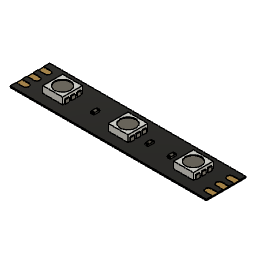
m v1 (Autodesk Fusion 360 design; units mm, degrees)
Autodesk Fusion 360 part; units mm, degrees
sketch "Sketch7" plane through (0, 0, 0) normal (0, 0, 1) x (1, 0, 0)
  line L0 (0, 0) -> (49.62, 0)
  line L1 (49.62, 0) -> (49.62, 10)
  line L2 (49.62, 10) -> (0, 10)
  line L3 (0, 10) -> (0, 0)
  line L4 (0, 10) -> (8.27, 10) construction
  line L5 (8.27, 10) -> (8.27, 0) construction
  line L6 (0, 5) -> (49.62, 5) construction
  line L7 (10.77, 2.5) -> (5.77, 2.5)
  line L8 (5.77, 2.5) -> (5.77, 7.5)
  line L9 (5.77, 7.5) -> (10.77, 7.5)
  line L10 (10.77, 7.5) -> (10.77, 2.5)
  line L11 (10.77, 2.5) -> (5.77, 7.5) construction
  line L12 (5.77, 2.5) -> (10.77, 7.5) construction
  line L13 (8.27, 5) -> (24.81, 5) construction
  line L14 (27.31, 2.5) -> (22.31, 2.5)
  line L15 (22.31, 2.5) -> (22.31, 7.5)
  line L16 (22.31, 7.5) -> (27.31, 7.5)
  line L17 (27.31, 7.5) -> (27.31, 2.5)
  line L18 (27.31, 2.5) -> (22.31, 7.5) construction
  line L19 (22.31, 2.5) -> (27.31, 7.5) construction
  line L20 (24.81, 5) -> (41.35, 5) construction
  line L21 (43.85, 2.5) -> (38.85, 2.5)
  line L22 (38.85, 2.5) -> (38.85, 7.5)
  line L23 (38.85, 7.5) -> (43.85, 7.5)
  line L24 (43.85, 7.5) -> (43.85, 2.5)
  line L25 (43.85, 2.5) -> (38.85, 7.5) construction
  line L26 (38.85, 2.5) -> (43.85, 7.5) construction
  point P0 (8.27, 5)
  point P1 (24.81, 5)
  point P2 (41.35, 5)
  dimension "d27" = 49.62
  dimension "d28" = 10
  dimension "d29" = 8.27
  dimension "d30" = 5
  dimension "d31" = 5
  dimension "d32" = 16.54
  dimension "d33" = 5
  dimension "d34" = 5
  dimension "d35" = 16.54
  dimension "d36" = 5
  dimension "d37" = 5
  constraint coincident L0.start L3.end
  constraint horizontal L0
  constraint perpendicular L0 L1
  constraint perpendicular L1 L2
  constraint perpendicular L0 L3
  constraint perpendicular L3 L4
  constraint coincident L0 L5.end
  constraint perpendicular L0 L5
  constraint midpoint L3 L6.start
  constraint midpoint L1 L6.end
  constraint horizontal L7
  constraint perpendicular L7 L8
  constraint parallel L7 L9
  constraint parallel L8 L10
  constraint coincident L11 P0
  constraint coincident L12 P0
  constraint midpoint L5 P0
  constraint coincident P0 L13.start
  constraint parallel L6 L13
  constraint horizontal L14
  constraint perpendicular L14 L15
  constraint parallel L14 L16
  constraint parallel L15 L17
  constraint coincident L18 P1
  constraint coincident L19 P1
  constraint coincident P1 L13.end
  constraint parallel L6 L20
  constraint horizontal L21
  constraint perpendicular L21 L22
  constraint parallel L21 L23
  constraint parallel L22 L24
  constraint coincident L25 P2
  constraint coincident L26 P2
  constraint coincident P2 L20.end
  measures "d27" distance of L0.start L0.end
  measures "d28" distance of L0.end L1.end
  measures "d29" distance of L2.end L4.end
  measures "d30" distance of L8.end L9.end
  measures "d31" distance of L7.end L8.end
  measures "d32" distance of P0 P1
  measures "d33" distance of L15.end L16.end
  measures "d34" distance of L14.end L15.end
  measures "d35" distance of P1 P2
  measures "d36" distance of L22.end L23.end
  measures "d37" distance of L21.end L22.end
extrude "Extrude4" add sketch "Sketch7" along normal blind 2 contours L7 L8 L9 L10 | L14 L15 L16 L17 | L21 L22 L23 L24 makes body 1 at (25.6433, 4.1667, 0) makes body 2 at (9.1033, 4.1667, 0) makes body 3 at (42.1833, 4.1667, 0)
extrude "Extrude3" add sketch "Sketch7" along normal blind 0.3 separate body makes body 4
sketch "Sketch8" plane through (0, 0, 2) normal (0, 0, 1) x (-1, 0, 0)
  line L0 (-10.77, -7.5) -> (-5.77, -7.5)
  line L1 (-5.77, -7.5) -> (-5.77, -2.5)
  line L2 (-5.77, -2.5) -> (-10.77, -2.5)
  line L3 (-10.77, -2.5) -> (-10.77, -7.5)
  circle A0 centre (-8.27, -5) radius 2
  circle A1 centre (-24.81, -5) radius 2
  circle A2 centre (-41.35, -5) radius 2
  point P0 (-8.27, -5)
  point P1 (-24.81, -5)
  point P2 (-41.35, -5)
  dimension "d42" = 4
  dimension "d43" = 4
  dimension "d44" = 4
  constraint coincident P0 A0.centre
  constraint coincident P1 A1.centre
  constraint coincident P2 A2.centre
  measures "d42" diameter of A0
  measures "d43" diameter of A1
  measures "d44" diameter of A2
extrude "Extrude5" cut sketch "Sketch8" against normal blind 0.2 contours A0 | A1 | A2 bodies 1 2 3
sketch "Sketch9" plane through (0, 0, 0.3) normal (0, 0, 1) x (-1, 0, 0)
  line L0 (-5.77, -7.5) -> (-10.77, -7.5)
  line L1 (-10.77, -7.5) -> (-10.77, -2.5)
  line L2 (-10.77, -2.5) -> (-5.77, -2.5)
  line L3 (-5.77, -2.5) -> (-5.77, -7.5)
  line L4 (-38.85, -7.5) -> (-43.85, -7.5)
  line L5 (-43.85, -7.5) -> (-43.85, -2.5)
  line L6 (-43.85, -2.5) -> (-38.85, -2.5)
  line L7 (-38.85, -2.5) -> (-38.85, -7.5)
  line L8 (-22.31, -7.5) -> (-27.31, -7.5)
  line L9 (-27.31, -7.5) -> (-27.31, -2.5)
  line L10 (-27.31, -2.5) -> (-22.31, -2.5)
  line L11 (-22.31, -2.5) -> (-22.31, -7.5)
  line L12 (0, -10) -> (0, 0)
  line L13 (0, 0) -> (-49.62, 0)
  line L14 (-49.62, 0) -> (-49.62, -10)
  line L15 (-49.62, -10) -> (0, -10)
  line L16 (-5.77, -7.5) -> (-5.77, -7) construction
  line L17 (-5.77, -7) -> (-5.77, -6)
  line L18 (-5.77, -6) -> (-5.77, -5.5) construction
  line L19 (-5.77, -5.5) -> (-5.77, -4.5)
  line L20 (-5.77, -4.5) -> (-5.77, -4) construction
  line L21 (-5.77, -4) -> (-5.77, -3) construction
  line L22 (-5.77, -3) -> (-5.77, -2.5) construction
  line L23 (-5.77, -7) -> (-5.57, -7)
  line L24 (-5.77, -6) -> (-5.57, -6)
  line L25 (-5.57, -6) -> (-5.57, -7)
  line L26 (-5.77, -5.5) -> (-5.57, -5.5)
  line L27 (-5.57, -5.5) -> (-5.57, -4.5)
  line L28 (-5.57, -4.5) -> (-5.77, -4.5)
  line L29 (-5.77, -3) -> (-5.57, -3)
  line L30 (-5.57, -3) -> (-5.57, -4)
  line L31 (-5.57, -4) -> (-5.77, -4)
  dimension "d47" = 0.5
  dimension "d48" = 1
  dimension "d49" = 0.5
  dimension "d50" = 1
  dimension "d51" = 0.5
  dimension "d52" = 1
  dimension "d53" = 0.2
  dimension "d54" = 0.2
  constraint coincident L0.start L3.end
  constraint perpendicular L0 L16
  constraint parallel L3 L17
  constraint parallel L3 L18
  constraint parallel L18 L19
  constraint parallel L3 L20
  constraint parallel L3 L21
  constraint coincident L2.end L3.start
  constraint perpendicular L16 L23
  constraint perpendicular L17 L24
  constraint perpendicular L18 L26
  constraint perpendicular L26 L27
  constraint perpendicular L22 L29
  constraint perpendicular L29 L30
  measures "d47" distance of L0.start L16.end
  measures "d48" distance of L16.end L17.end
  measures "d49" distance of L17.end L18.end
  measures "d50" distance of L18.end L19.end
  measures "d51" distance of L19.end L20.end
  measures "d52" distance of L20.end L21.end
  measures "d53" distance of L16.end L23.end
  measures "d54" distance of L17.end L24.end
extrude "Extrude6" add sketch "Sketch9" along normal blind 1 contours L3 L17 L23 L24 L25 | L3 L19 L26 L27 L28 | L3 L29 L30 L31 bodies 2 4
sketch "Sketch10" plane through (0, 0, 0.3) normal (0, 0, 1) x (-1, 0, 0)
  line L0 (-5.77, -6) -> (-5.57, -6)
  line L1 (-5.57, -6) -> (-5.57, -7)
  line L2 (-5.57, -7) -> (-5.77, -7)
  line L3 (-5.77, -7) -> (-5.77, -7.5)
  line L4 (-5.77, -7.5) -> (-10.77, -7.5)
  line L5 (-10.77, -7.5) -> (-10.77, -2.5)
  line L6 (-10.77, -2.5) -> (-5.77, -2.5)
  line L7 (-5.77, -2.5) -> (-5.77, -3)
  line L8 (-5.77, -3) -> (-5.57, -3)
  line L9 (-5.57, -3) -> (-5.57, -4)
  line L10 (-5.57, -4) -> (-5.77, -4)
  line L11 (-5.77, -4) -> (-5.77, -4.5)
  line L12 (-5.77, -4.5) -> (-5.57, -4.5)
  line L13 (-5.57, -4.5) -> (-5.57, -5.5)
  line L14 (-5.57, -5.5) -> (-5.77, -5.5)
  line L15 (-5.77, -5.5) -> (-5.77, -6)
  line L16 (-38.85, -7.5) -> (-43.85, -7.5)
  line L17 (-43.85, -7.5) -> (-43.85, -2.5)
  line L18 (-43.85, -2.5) -> (-38.85, -2.5)
  line L19 (-38.85, -2.5) -> (-38.85, -7.5)
  line L20 (-22.31, -7.5) -> (-27.31, -7.5)
  line L21 (-27.31, -7.5) -> (-27.31, -2.5)
  line L22 (-27.31, -2.5) -> (-22.31, -2.5)
  line L23 (-22.31, -2.5) -> (-22.31, -7.5)
  line L24 (0, -10) -> (0, 0)
  line L25 (0, 0) -> (-49.62, 0)
  line L26 (-49.62, 0) -> (-49.62, -10)
  line L27 (-49.62, -10) -> (0, -10)
  line L28 (-5.77, -6) -> (-10.77, -6) construction
  line L29 (-5.77, -4.5) -> (-10.77, -4.5) construction
  line L30 (-5.77, -3) -> (-10.77, -3) construction
  line L31 (-5.77, -4) -> (-10.77, -4) construction
  line L32 (-5.77, -5.5) -> (-10.77, -5.5) construction
  line L33 (-5.77, -7) -> (-10.77, -7) construction
  line L34 (-10.77, -7) -> (-10.97, -7)
  line L35 (-10.97, -7) -> (-10.97, -3) construction
  line L36 (-10.97, -3) -> (-10.77, -3)
  line L37 (-10.77, -4) -> (-10.97, -4)
  line L38 (-10.97, -4) -> (-10.97, -3)
  line L39 (-10.77, -4.5) -> (-10.97, -4.5)
  line L40 (-10.97, -4.5) -> (-10.97, -5.5)
  line L41 (-10.77, -5.5) -> (-10.97, -5.5)
  line L42 (-10.77, -6) -> (-10.97, -6)
  line L43 (-10.97, -6) -> (-10.97, -7)
  line L44 (-10.97, -3) -> (-43.85, -3) construction
  line L45 (-43.85, -3) -> (-44.05, -3) construction
  line L46 (-10.97, -4) -> (-43.85, -4) construction
  line L47 (-44.05, -7) -> (-10.77, -7) construction
  line L48 (-10.97, -6) -> (-44.8, -6) construction
  line L49 (-10.97, -5.5) -> (-44.05, -5.5) construction
  line L50 (-10.77, -4.5) -> (-44.05, -4.5) construction
  line L51 (-22.31, -3) -> (-22.11, -3) construction
  line L52 (-22.11, -3) -> (-22.11, -7) construction
  line L53 (-27.31, -7) -> (-27.51, -7) construction
  line L54 (-27.51, -7) -> (-27.51, -3) construction
  line L55 (-27.31, -3) -> (-27.51, -3) construction
  line L56 (-43.85, -7) -> (-44.05, -7)
  line L57 (-43.85, -7) -> (-43.85, -3)
  line L58 (-43.85, -3) -> (-44.05, -3)
  line L59 (-43.85, -4) -> (-44.05, -4)
  line L60 (-43.85, -4.5) -> (-44.05, -4.5)
  line L61 (-43.85, -5.5) -> (-44.05, -5.5)
  line L62 (-43.85, -6.004) -> (-44.05, -6)
  line L63 (-38.85, -3) -> (-38.65, -3)
  line L64 (-38.65, -7) -> (-38.85, -7)
  line L65 (-38.85, -3) -> (-38.85, -7)
  line L66 (-38.65, -6) -> (-38.85, -6)
  line L67 (-38.65, -5.5) -> (-38.85, -5.5)
  line L68 (-38.65, -4.5) -> (-38.85, -4.5028)
  line L69 (-38.65, -4) -> (-38.85, -3.9993)
  line L70 (-38.65, -3) -> (-38.65, -4)
  line L71 (-38.65, -4.5) -> (-38.65, -5.5)
  line L72 (-38.65, -6) -> (-38.65, -7)
  line L73 (-44.05, -3) -> (-44.05, -4)
  line L74 (-44.05, -4.5) -> (-44.05, -5.5)
  line L75 (-44.05, -6) -> (-44.05, -7)
  line L76 (-27.31, -3) -> (-27.51, -3)
  line L77 (-27.51, -3) -> (-27.51, -4)
  line L78 (-27.51, -4) -> (-27.31, -4)
  line L79 (-27.31, -4.5) -> (-27.51, -4.5)
  line L80 (-27.51, -4.5) -> (-27.51, -5.5)
  line L81 (-27.51, -5.5) -> (-27.3, -5.5)
  line L82 (-27.31, -6) -> (-27.51, -6)
  line L83 (-27.51, -6) -> (-27.51, -7)
  line L84 (-27.51, -7) -> (-27.31, -7)
  line L85 (-22.31, -7) -> (-22.11, -7)
  line L86 (-22.11, -6) -> (-22.11, -7)
  line L87 (-22.11, -6) -> (-22.31, -6)
  line L88 (-22.11, -5.5) -> (-22.31, -5.5)
  line L89 (-22.11, -5.5) -> (-22.11, -4.5)
  line L90 (-22.31, -4.5) -> (-22.11, -4.5)
  line L91 (-22.11, -4) -> (-22.31, -4)
  line L92 (-22.11, -4) -> (-22.11, -3)
  line L93 (-22.11, -3) -> (-22.31, -3)
  dimension "d57" = 0.2
  dimension "d60" = 32.88
  dimension "d61" = 0.2
  dimension "d62" = 4
  dimension "d63" = 0.2
  dimension "d64" = 0.2
  dimension "d65" = 0.2
  constraint coincident L0.start L15.end
  constraint coincident L5 L28.end
  constraint perpendicular L5 L28
  constraint coincident L11.end L12.start
  constraint coincident L5 L29.end
  constraint perpendicular L5 L29
  constraint coincident L7.end L8.start
  constraint coincident L5 L30.end
  constraint perpendicular L5 L30
  constraint coincident L10.end L11.start
  constraint coincident L5 L31.end
  constraint perpendicular L5 L31
  constraint coincident L14.end L15.start
  constraint coincident L5 L32.end
  constraint perpendicular L5 L32
  constraint coincident L2.end L3.start
  constraint coincident L5 L33.end
  constraint perpendicular L5 L33
  constraint perpendicular L5 L34
  constraint perpendicular L34 L35
  constraint coincident L35 L37.end
  constraint perpendicular L35 L37
  constraint coincident L35 L39.end
  constraint perpendicular L35 L39
  constraint coincident L35 L40.end
  constraint coincident L35 L42.end
  constraint perpendicular L35 L42
  constraint coincident L17 L44.end
  constraint perpendicular L17 L44
  constraint horizontal L45
  constraint coincident L17 L46.end
  constraint perpendicular L17 L46
  constraint perpendicular L17 L48
  constraint coincident L44 L51.start
  constraint coincident L23 L51.start
  constraint perpendicular L23 L51
  constraint coincident L47 L52.end
  constraint perpendicular L47 L52
  constraint coincident L47 L53.start
  constraint coincident L21 L53.start
  constraint perpendicular L21 L53
  constraint coincident L44 L54.end
  constraint perpendicular L44 L54
  constraint coincident L44 L55.start
  constraint coincident L21 L55.start
  constraint coincident L47 L56.start
  constraint coincident L17 L56.start
  constraint coincident L57 L60.start
  constraint coincident L50 L60.start
  constraint coincident L57 L61.start
  constraint coincident L49 L61.start
  constraint coincident L57 L62.start
  constraint coincident L48 L62.end
  constraint coincident L44 L63.start
  constraint coincident L19 L63.start
  constraint perpendicular L19 L63
  constraint coincident L47 L64.start
  constraint coincident L47 L64.end
  constraint coincident L19 L64.end
  constraint coincident L48 L66.start
  constraint coincident L48 L66.end
  constraint coincident L19 L66.end
  constraint coincident L49 L67.start
  constraint coincident L65 L67.end
  constraint coincident L49 L67.end
  constraint coincident L50 L68.start
  constraint coincident L65 L68.end
  constraint coincident L46 L69.start
  constraint coincident L65 L69.end
  constraint parallel L70 L71
  constraint perpendicular L64 L72
  constraint perpendicular L59 L73
  constraint perpendicular L61 L74
  constraint parallel L74 L75
  constraint coincident L54 L77.end
  constraint coincident L46 L77.end
  constraint coincident L46 L78.end
  constraint coincident L21 L78.end
  constraint coincident L50 L79.start
  constraint coincident L21 L79.start
  constraint coincident L54 L79.end
  constraint coincident L50 L79.end
  constraint perpendicular L54 L79
  constraint midpoint L49 L80.end
  constraint perpendicular L49 L80
  constraint coincident L49 L81.end
  constraint perpendicular L80 L81
  constraint coincident L48 L82.start
  constraint coincident L21 L82.start
  constraint coincident L54 L82.end
  constraint coincident L48 L82.end
  constraint coincident L47 L85.start
  constraint coincident L23 L85.start
  constraint coincident L52 L86.start
  constraint coincident L48 L86.start
  constraint coincident L48 L87.end
  constraint coincident L23 L87.end
  constraint coincident L52 L88.start
  constraint coincident L49 L88.start
  constraint coincident L49 L88.end
  constraint coincident L23 L88.end
  constraint perpendicular L23 L88
  constraint coincident L52 L89.end
  constraint coincident L50 L89.end
  constraint coincident L50 L90.start
  constraint coincident L23 L90.start
  constraint perpendicular L89 L90
  constraint coincident L46 L91.start
  constraint coincident L52 L91.start
  constraint coincident L46 L91.end
  constraint coincident L23 L91.end
  measures "d57" distance of L33.end L34.end
  measures "d60" distance of L35.end L44.end
  measures "d61" distance of L44.end L45.end
  measures "d62" distance of L45.end L47.start
  measures "d63" distance of L51.start L51.end
  measures "d64" distance of L53.start L53.end
  measures "d65" distance of L63.start L63.end
extrude "Extrude7" add sketch "Sketch10" along normal blind 1 contours L5 L34 L42 L43 | L5 L39 L40 L41 | L5 L36 L37 L38 | L19 L64 L65 L66 L72 | L17 L56 L57 L62 L75 | L19 L65 L67 L68 L71 | L17 L57 L60 L61 L74 | L19 L63 L65 L69 L70 | L17 L57 L58 L59 L73 | L23 L85 L86 L87 | L21 L82 L83 L84 | L23 L88 L89 L90 | L21 L79 L80 L81 | L23 L91 L92 L93 | L21 L76 L77 L78 bodies 1 2 3
sketch "Sketch11" plane through (0, 0, 0.3) normal (0, 0, 1) x (-1, 0, 0)
  line L0 (-44.05, -3) -> (-43.85, -3)
  line L1 (-43.85, -3) -> (-43.85, -2.5)
  line L2 (-43.85, -2.5) -> (-38.85, -2.5)
  line L3 (-38.85, -2.5) -> (-38.85, -3)
  line L4 (-38.85, -3) -> (-38.65, -3)
  line L5 (-38.65, -3) -> (-38.65, -4)
  line L6 (-38.65, -4) -> (-38.85, -3.9993)
  line L7 (-38.85, -3.9993) -> (-38.85, -4.5028)
  line L8 (-38.85, -4.5028) -> (-38.65, -4.5)
  line L9 (-38.65, -4.5) -> (-38.65, -5.5)
  line L10 (-38.65, -5.5) -> (-38.85, -5.5)
  line L11 (-38.85, -5.5) -> (-38.85, -6)
  line L12 (-38.85, -6) -> (-38.65, -6)
  line L13 (-38.65, -6) -> (-38.65, -7)
  line L14 (-38.65, -7) -> (-38.85, -7)
  line L15 (-38.85, -7) -> (-38.85, -7.5)
  line L16 (-38.85, -7.5) -> (-43.85, -7.5)
  line L17 (-43.85, -7.5) -> (-43.85, -7)
  line L18 (-43.85, -7) -> (-44.05, -7)
  line L19 (-44.05, -7) -> (-44.05, -6)
  line L20 (-44.05, -6) -> (-43.85, -6.004)
  line L21 (-43.85, -6.004) -> (-43.85, -5.5)
  line L22 (-43.85, -5.5) -> (-44.05, -5.5)
  line L23 (-44.05, -5.5) -> (-44.05, -4.5)
  line L24 (-44.05, -4.5) -> (-43.85, -4.5)
  line L25 (-43.85, -4.5) -> (-43.85, -4)
  line L26 (-43.85, -4) -> (-44.05, -4)
  line L27 (-44.05, -4) -> (-44.05, -3)
  line L28 (-27.51, -6) -> (-27.31, -6)
  line L29 (-27.31, -6) -> (-27.31, -5.5)
  line L30 (-27.31, -5.5) -> (-27.51, -5.5)
  line L31 (-27.51, -5.5) -> (-27.51, -4.5)
  line L32 (-27.51, -4.5) -> (-27.31, -4.5)
  line L33 (-27.31, -4.5) -> (-27.31, -4)
  line L34 (-27.31, -4) -> (-27.51, -4)
  line L35 (-27.51, -4) -> (-27.51, -3)
  line L36 (-27.51, -3) -> (-27.31, -3)
  line L37 (-27.31, -3) -> (-27.31, -2.5)
  line L38 (-27.31, -2.5) -> (-22.31, -2.5)
  line L39 (-22.31, -2.5) -> (-22.31, -3)
  line L40 (-22.31, -3) -> (-22.11, -3)
  line L41 (-22.11, -3) -> (-22.11, -4)
  line L42 (-22.11, -4) -> (-22.31, -4)
  line L43 (-22.31, -4) -> (-22.31, -4.5)
  line L44 (-22.31, -4.5) -> (-22.11, -4.5)
  line L45 (-22.11, -4.5) -> (-22.11, -5.5)
  line L46 (-22.11, -5.5) -> (-22.31, -5.5)
  line L47 (-22.31, -5.5) -> (-22.31, -6)
  line L48 (-22.31, -6) -> (-22.11, -6)
  line L49 (-22.11, -6) -> (-22.11, -7)
  line L50 (-22.11, -7) -> (-22.31, -7)
  line L51 (-22.31, -7) -> (-22.31, -7.5)
  line L52 (-22.31, -7.5) -> (-27.31, -7.5)
  line L53 (-27.31, -7.5) -> (-27.31, -7)
  line L54 (-27.31, -7) -> (-27.51, -7)
  line L55 (-27.51, -7) -> (-27.51, -6)
  line L56 (0, -10) -> (0, 0)
  line L57 (0, 0) -> (-49.62, 0)
  line L58 (-49.62, 0) -> (-49.62, -10)
  line L59 (-49.62, -10) -> (0, -10)
  line L60 (-10.77, -5.5) -> (-10.97, -5.5)
  line L61 (-10.97, -5.5) -> (-10.97, -4.5)
  line L62 (-10.97, -4.5) -> (-10.77, -4.5)
  line L63 (-10.77, -4.5) -> (-10.77, -4)
  line L64 (-10.77, -4) -> (-10.97, -4)
  line L65 (-10.97, -4) -> (-10.97, -3)
  line L66 (-10.97, -3) -> (-10.77, -3)
  line L67 (-10.77, -3) -> (-10.77, -2.5)
  line L68 (-10.77, -2.5) -> (-5.77, -2.5)
  line L69 (-5.77, -2.5) -> (-5.77, -3)
  line L70 (-5.77, -3) -> (-5.57, -3)
  line L71 (-5.57, -3) -> (-5.57, -4)
  line L72 (-5.57, -4) -> (-5.77, -4)
  line L73 (-5.77, -4) -> (-5.77, -4.5)
  line L74 (-5.77, -4.5) -> (-5.57, -4.5)
  line L75 (-5.57, -4.5) -> (-5.57, -5.5)
  line L76 (-5.57, -5.5) -> (-5.77, -5.5)
  line L77 (-5.77, -5.5) -> (-5.77, -6)
  line L78 (-5.77, -6) -> (-5.57, -6)
  line L79 (-5.57, -6) -> (-5.57, -7)
  line L80 (-5.57, -7) -> (-5.77, -7)
  line L81 (-5.77, -7) -> (-5.77, -7.5)
  line L82 (-5.77, -7.5) -> (-10.77, -7.5)
  line L83 (-10.77, -7.5) -> (-10.77, -7)
  line L84 (-10.77, -7) -> (-10.97, -7)
  line L85 (-10.97, -7) -> (-10.97, -6)
  line L86 (-10.97, -6) -> (-10.77, -6)
  line L87 (-10.77, -6) -> (-10.77, -5.5)
  line L88 (0, -5) -> (0, -5.75)
  line L89 (0, -5) -> (0, -4.25)
  line L90 (0, -4.25) -> (-2.5, -4.25)
  line L91 (-2.5, -4.25) -> (-2.5, -5.75)
  line L92 (-2.5, -5.75) -> (0, -5.75)
  line L93 (0, -4.25) -> (0, -3) construction
  line L94 (0, -3) -> (0, -1.5) construction
  line L95 (0, -1.5) -> (-2.5, -1.5)
  line L96 (-2.5, -1.5) -> (-2.5, -3)
  line L97 (-2.5, -3) -> (0, -3)
  line L98 (0, -5.75) -> (0, -7) construction
  line L99 (0, -7) -> (-2.5, -7)
  line L100 (-2.5, -7) -> (-2.5, -8.5)
  line L101 (-2.5, -8.5) -> (0, -8.5)
  line L102 (-2.5, -1.5) -> (-1.5, -1.5)
  line L103 (-2.5, -1.5) -> (-1.75, -1.5) construction
  line L104 (-1.75, -1.5) -> (-1.75, -3) construction
  circle A0 centre (-1.75, -2.25) radius 0.75
  line L105 (-1.75, -3) -> (-1.75, -8.5) construction
  line L106 (-1.75, -4.25) -> (-1.75, -5.75) construction
  line L107 (-1.75, -7) -> (-1.75, -8.5) construction
  circle A1 centre (-1.75, -5) radius 0.75
  circle A2 centre (-1.75, -7.75) radius 0.75
  dimension "d66" = 0.75
  dimension "d67" = 0.75
  dimension "d68" = 1.5
  dimension "d69" = 1.5
  dimension "d72" = 1
  dimension "d73" = 0.75
  dimension "d74" = 1.5
  dimension "d75" = 1.5
  dimension "d76" = 1.5
  constraint midpoint L56 L88.start
  constraint parallel L56 L88
  constraint parallel L88 L89
  constraint perpendicular L89 L90
  constraint perpendicular L90 L91
  constraint coincident L56 L93.end
  constraint perpendicular L90 L93
  constraint parallel L56 L94
  constraint perpendicular L94 L95
  constraint perpendicular L95 L96
  constraint perpendicular L93 L97
  constraint coincident L56 L98.end
  constraint perpendicular L56 L99
  constraint perpendicular L99 L100
  constraint coincident L56 L101.end
  constraint perpendicular L100 L101
  constraint perpendicular L96 L102
  constraint perpendicular L96 L103
  constraint coincident L97 L104.end
  constraint perpendicular L97 L104
  constraint midpoint L104 A0.centre
  constraint coincident L101 L105.end
  constraint perpendicular L101 L105
  constraint coincident L105 L106.start
  constraint coincident L90 L106.start
  constraint midpoint L105 L106.end
  constraint coincident L105 L107.start
  constraint coincident L99 L107.start
  constraint perpendicular L101 L107
  constraint midpoint L106 A1.centre
  constraint midpoint L107 A2.centre
  measures "d66" distance of L88.start L88.end
  measures "d67" distance of L88.start L89.end
  measures "d68" distance of L90.end L91.end
  measures "d69" distance of L93.end L94.end
  measures "d72" distance of L95.end L102.end
  measures "d73" distance of L95.end L103.end
  measures "d74" diameter of A0
  measures "d75" diameter of A1
  measures "d76" diameter of A2
sketch "Sketch13" plane through (0, 0, 0.3) normal (0, 0, 1) x (-1, 0, 0)
  line L0 (0, 0) -> (-49.62, 0)
  line L1 (-49.62, 0) -> (-49.62, -10)
  line L2 (-49.62, -10) -> (0, -10)
  line L3 (0, -10) -> (0, 0)
  line L4 (-44.05, -3) -> (-43.85, -3)
  line L5 (-43.85, -3) -> (-43.85, -2.5)
  line L6 (-43.85, -2.5) -> (-38.85, -2.5)
  line L7 (-38.85, -2.5) -> (-38.85, -3)
  line L8 (-38.85, -3) -> (-38.65, -3)
  line L9 (-38.65, -3) -> (-38.65, -4)
  line L10 (-38.65, -4) -> (-38.85, -3.9993)
  line L11 (-38.85, -3.9993) -> (-38.85, -4.5028)
  line L12 (-38.85, -4.5028) -> (-38.65, -4.5)
  line L13 (-38.65, -4.5) -> (-38.65, -5.5)
  line L14 (-38.65, -5.5) -> (-38.85, -5.5)
  line L15 (-38.85, -5.5) -> (-38.85, -6)
  line L16 (-38.85, -6) -> (-38.65, -6)
  line L17 (-38.65, -6) -> (-38.65, -7)
  line L18 (-38.65, -7) -> (-38.85, -7)
  line L19 (-38.85, -7) -> (-38.85, -7.5)
  line L20 (-38.85, -7.5) -> (-43.85, -7.5)
  line L21 (-43.85, -7.5) -> (-43.85, -7)
  line L22 (-43.85, -7) -> (-44.05, -7)
  line L23 (-44.05, -7) -> (-44.05, -6)
  line L24 (-44.05, -6) -> (-43.85, -6.004)
  line L25 (-43.85, -6.004) -> (-43.85, -5.5)
  line L26 (-43.85, -5.5) -> (-44.05, -5.5)
  line L27 (-44.05, -5.5) -> (-44.05, -4.5)
  line L28 (-44.05, -4.5) -> (-43.85, -4.5)
  line L29 (-43.85, -4.5) -> (-43.85, -4)
  line L30 (-43.85, -4) -> (-44.05, -4)
  line L31 (-44.05, -4) -> (-44.05, -3)
  line L32 (-27.51, -6) -> (-27.31, -6)
  line L33 (-27.31, -6) -> (-27.31, -5.5)
  line L34 (-27.31, -5.5) -> (-27.51, -5.5)
  line L35 (-27.51, -5.5) -> (-27.51, -4.5)
  line L36 (-27.51, -4.5) -> (-27.31, -4.5)
  line L37 (-27.31, -4.5) -> (-27.31, -4)
  line L38 (-27.31, -4) -> (-27.51, -4)
  line L39 (-27.51, -4) -> (-27.51, -3)
  line L40 (-27.51, -3) -> (-27.31, -3)
  line L41 (-27.31, -3) -> (-27.31, -2.5)
  line L42 (-27.31, -2.5) -> (-22.31, -2.5)
  line L43 (-22.31, -2.5) -> (-22.31, -3)
  line L44 (-22.31, -3) -> (-22.11, -3)
  line L45 (-22.11, -3) -> (-22.11, -4)
  line L46 (-22.11, -4) -> (-22.31, -4)
  line L47 (-22.31, -4) -> (-22.31, -4.5)
  line L48 (-22.31, -4.5) -> (-22.11, -4.5)
  line L49 (-22.11, -4.5) -> (-22.11, -5.5)
  line L50 (-22.11, -5.5) -> (-22.31, -5.5)
  line L51 (-22.31, -5.5) -> (-22.31, -6)
  line L52 (-22.31, -6) -> (-22.11, -6)
  line L53 (-22.11, -6) -> (-22.11, -7)
  line L54 (-22.11, -7) -> (-22.31, -7)
  line L55 (-22.31, -7) -> (-22.31, -7.5)
  line L56 (-22.31, -7.5) -> (-27.31, -7.5)
  line L57 (-27.31, -7.5) -> (-27.31, -7)
  line L58 (-27.31, -7) -> (-27.51, -7)
  line L59 (-27.51, -7) -> (-27.51, -6)
  line L60 (-10.77, -5.5) -> (-10.97, -5.5)
  line L61 (-10.97, -5.5) -> (-10.97, -4.5)
  line L62 (-10.97, -4.5) -> (-10.77, -4.5)
  line L63 (-10.77, -4.5) -> (-10.77, -4)
  line L64 (-10.77, -4) -> (-10.97, -4)
  line L65 (-10.97, -4) -> (-10.97, -3)
  line L66 (-10.97, -3) -> (-10.77, -3)
  line L67 (-10.77, -3) -> (-10.77, -2.5)
  line L68 (-10.77, -2.5) -> (-5.77, -2.5)
  line L69 (-5.77, -2.5) -> (-5.77, -3)
  line L70 (-5.77, -3) -> (-5.57, -3)
  line L71 (-5.57, -3) -> (-5.57, -4)
  line L72 (-5.57, -4) -> (-5.77, -4)
  line L73 (-5.77, -4) -> (-5.77, -4.5)
  line L74 (-5.77, -4.5) -> (-5.57, -4.5)
  line L75 (-5.57, -4.5) -> (-5.57, -5.5)
  line L76 (-5.57, -5.5) -> (-5.77, -5.5)
  line L77 (-5.77, -5.5) -> (-5.77, -6)
  line L78 (-5.77, -6) -> (-5.57, -6)
  line L79 (-5.57, -6) -> (-5.57, -7)
  line L80 (-5.57, -7) -> (-5.77, -7)
  line L81 (-5.77, -7) -> (-5.77, -7.5)
  line L82 (-5.77, -7.5) -> (-10.77, -7.5)
  line L83 (-10.77, -7.5) -> (-10.77, -7)
  line L84 (-10.77, -7) -> (-10.97, -7)
  line L85 (-10.97, -7) -> (-10.97, -6)
  line L86 (-10.97, -6) -> (-10.77, -6)
  line L87 (-10.77, -6) -> (-10.77, -5.5)
  line L88 (-49.62, -5) -> (-49.62, -4.25)
  line L89 (-49.62, -5) -> (-49.62, -5.75)
  line L90 (-49.62, -5.75) -> (-47.12, -5.75)
  line L91 (-47.12, -5.75) -> (-47.12, -4.25)
  line L92 (-47.12, -4.25) -> (-49.62, -4.25)
  line L93 (-49.62, -4.25) -> (-49.62, -3) construction
  line L94 (-49.62, -3) -> (-47.12, -3)
  line L95 (-47.12, -3) -> (-47.12, -1.5)
  line L96 (-47.12, -1.5) -> (-49.62, -1.5)
  line L97 (-49.62, -5.75) -> (-49.62, -7) construction
  line L98 (-49.62, -7) -> (-47.12, -7)
  line L99 (-47.12, -7) -> (-47.12, -8.5)
  line L100 (-47.12, -8.5) -> (-49.62, -8.5)
  line L101 (-47.12, -8.5) -> (-47.87, -8.5) construction
  line L102 (-47.87, -8.5) -> (-47.87, -1.5) construction
  line L103 (-47.87, -8.5) -> (-47.87, -7) construction
  line L104 (-47.87, -5.75) -> (-47.87, -4.4) construction
  line L105 (-47.87, -3) -> (-47.87, -1.5) construction
  circle A0 centre (-47.87, -7.75) radius 0.75
  circle A1 centre (-47.87, -5) radius 0.75
  circle A2 centre (-47.87, -2.25) radius 0.75
  dimension "d77" = 0.75
  dimension "d78" = 0.75
  dimension "d79" = 2.5
  dimension "d80" = 1.5
  dimension "d81" = 1.25
  dimension "d82" = 2.5
  dimension "d83" = 1.5
  dimension "d84" = 1.25
  dimension "d85" = 2.5
  dimension "d86" = 1.5
  dimension "d87" = 0.75
  dimension "d88" = 1.5
  dimension "d89" = 1.5
  dimension "d90" = 1.5
  constraint midpoint L1 L88.start
  constraint parallel L1 L88
  constraint parallel L1 L89
  constraint perpendicular L1 L90
  constraint perpendicular L90 L91
  constraint perpendicular L92 L93
  constraint perpendicular L93 L94
  constraint perpendicular L94 L95
  constraint coincident L1 L96.end
  constraint perpendicular L1 L96
  constraint perpendicular L90 L97
  constraint perpendicular L97 L98
  constraint perpendicular L98 L99
  constraint coincident L1 L100.end
  constraint perpendicular L1 L100
  constraint perpendicular L99 L101
  constraint coincident L96 L102.end
  constraint perpendicular L96 L102
  constraint coincident L98 L103.end
  constraint coincident L102 L103.end
  constraint coincident L90 L104.start
  constraint coincident L102 L104.start
  constraint coincident L102 L104.end
  constraint perpendicular L90 L104
  constraint coincident L102 L105.start
  constraint coincident L94 L105.start
  constraint midpoint L103 A0.centre
  constraint midpoint L102 A1.centre
  constraint midpoint L105 A2.centre
  measures "d77" distance of L88.start L88.end
  measures "d78" distance of L88.start L89.end
  measures "d79" distance of L89.end L90.end
  measures "d80" distance of L90.end L91.end
  measures "d81" distance of L88.end L93.end
  measures "d82" distance of L93.end L94.end
  measures "d83" distance of L94.end L95.end
  measures "d84" distance of L89.end L97.end
  measures "d85" distance of L97.end L98.end
  measures "d86" distance of L98.end L99.end
  measures "d87" distance of L99.end L101.end
  measures "d88" diameter of A0
  measures "d89" diameter of A1
  measures "d90" diameter of A2
extrude "Extrude8" cut sketch "Sketch11" sketch "Sketch13" against normal blind 0.1 contours L56 L99 L101 A2 | A2 | L56 L88 L89 L90 L92 A1 | A1 | L56 L95 L97 L102 A0 | A0 of sketch 2 contours L1 L94 L96 A2 | A2 | L1 L98 L100 A0 | L1 L88 L89 L90 L92 A1 | A0 | A1 bodies 1
sketch "Sketch14" plane through (0, 0, 0.3) normal (0, 0, 1) x (-1, 0, 0)
  line L0 (-10.77, -5.5) -> (-10.97, -5.5)
  line L1 (-10.97, -5.5) -> (-10.97, -4.5)
  line L2 (-10.97, -4.5) -> (-10.77, -4.5)
  line L3 (-10.77, -4.5) -> (-10.77, -4)
  line L4 (-10.77, -4) -> (-10.97, -4)
  line L5 (-10.97, -4) -> (-10.97, -3)
  line L6 (-10.97, -3) -> (-10.77, -3)
  line L7 (-10.77, -3) -> (-10.77, -2.5)
  line L8 (-10.77, -2.5) -> (-5.77, -2.5)
  line L9 (-5.77, -2.5) -> (-5.77, -3)
  line L10 (-5.77, -3) -> (-5.57, -3)
  line L11 (-5.57, -3) -> (-5.57, -4)
  line L12 (-5.57, -4) -> (-5.77, -4)
  line L13 (-5.77, -4) -> (-5.77, -4.5)
  line L14 (-5.77, -4.5) -> (-5.57, -4.5)
  line L15 (-5.57, -4.5) -> (-5.57, -5.5)
  line L16 (-5.57, -5.5) -> (-5.77, -5.5)
  line L17 (-5.77, -5.5) -> (-5.77, -6)
  line L18 (-5.77, -6) -> (-5.57, -6)
  line L19 (-5.57, -6) -> (-5.57, -7)
  line L20 (-5.57, -7) -> (-5.77, -7)
  line L21 (-5.77, -7) -> (-5.77, -7.5)
  line L22 (-5.77, -7.5) -> (-10.77, -7.5)
  line L23 (-10.77, -7.5) -> (-10.77, -7)
  line L24 (-10.77, -7) -> (-10.97, -7)
  line L25 (-10.97, -7) -> (-10.97, -6)
  line L26 (-10.97, -6) -> (-10.77, -6)
  line L27 (-10.77, -6) -> (-10.77, -5.5)
  line L28 (-27.51, -6) -> (-27.31, -6)
  line L29 (-27.31, -6) -> (-27.31, -5.5)
  line L30 (-27.31, -5.5) -> (-27.51, -5.5)
  line L31 (-27.51, -5.5) -> (-27.51, -4.5)
  line L32 (-27.51, -4.5) -> (-27.31, -4.5)
  line L33 (-27.31, -4.5) -> (-27.31, -4)
  line L34 (-27.31, -4) -> (-27.51, -4)
  line L35 (-27.51, -4) -> (-27.51, -3)
  line L36 (-27.51, -3) -> (-27.31, -3)
  line L37 (-27.31, -3) -> (-27.31, -2.5)
  line L38 (-27.31, -2.5) -> (-22.31, -2.5)
  line L39 (-22.31, -2.5) -> (-22.31, -3)
  line L40 (-22.31, -3) -> (-22.11, -3)
  line L41 (-22.11, -3) -> (-22.11, -4)
  line L42 (-22.11, -4) -> (-22.31, -4)
  line L43 (-22.31, -4) -> (-22.31, -4.5)
  line L44 (-22.31, -4.5) -> (-22.11, -4.5)
  line L45 (-22.11, -4.5) -> (-22.11, -5.5)
  line L46 (-22.11, -5.5) -> (-22.31, -5.5)
  line L47 (-22.31, -5.5) -> (-22.31, -6)
  line L48 (-22.31, -6) -> (-22.11, -6)
  line L49 (-22.11, -6) -> (-22.11, -7)
  line L50 (-22.11, -7) -> (-22.31, -7)
  line L51 (-22.31, -7) -> (-22.31, -7.5)
  line L52 (-22.31, -7.5) -> (-27.31, -7.5)
  line L53 (-27.31, -7.5) -> (-27.31, -7)
  line L54 (-27.31, -7) -> (-27.51, -7)
  line L55 (-27.51, -7) -> (-27.51, -6)
  line L56 (-44.05, -3) -> (-43.85, -3)
  line L57 (-43.85, -3) -> (-43.85, -2.5)
  line L58 (-43.85, -2.5) -> (-38.85, -2.5)
  line L59 (-38.85, -2.5) -> (-38.85, -3)
  line L60 (-38.85, -3) -> (-38.65, -3)
  line L61 (-38.65, -3) -> (-38.65, -4)
  line L62 (-38.65, -4) -> (-38.85, -3.9993)
  line L63 (-38.85, -3.9993) -> (-38.85, -4.5028)
  line L64 (-38.85, -4.5028) -> (-38.65, -4.5)
  line L65 (-38.65, -4.5) -> (-38.65, -5.5)
  line L66 (-38.65, -5.5) -> (-38.85, -5.5)
  line L67 (-38.85, -5.5) -> (-38.85, -6)
  line L68 (-38.85, -6) -> (-38.65, -6)
  line L69 (-38.65, -6) -> (-38.65, -7)
  line L70 (-38.65, -7) -> (-38.85, -7)
  line L71 (-38.85, -7) -> (-38.85, -7.5)
  line L72 (-38.85, -7.5) -> (-43.85, -7.5)
  line L73 (-43.85, -7.5) -> (-43.85, -7)
  line L74 (-43.85, -7) -> (-44.05, -7)
  line L75 (-44.05, -7) -> (-44.05, -6)
  line L76 (-44.05, -6) -> (-43.85, -6.004)
  line L77 (-43.85, -6.004) -> (-43.85, -5.5)
  line L78 (-43.85, -5.5) -> (-44.05, -5.5)
  line L79 (-44.05, -5.5) -> (-44.05, -4.5)
  line L80 (-44.05, -4.5) -> (-43.85, -4.5)
  line L81 (-43.85, -4.5) -> (-43.85, -4)
  line L82 (-43.85, -4) -> (-44.05, -4)
  line L83 (-44.05, -4) -> (-44.05, -3)
  line L84 (-49.62, -4.25) -> (-47.87, -4.25)
  arc A0 (-47.87, -5.75) -> (-47.87, -4.25) centre (-47.87, -5) ccw
  line L85 (-47.87, -5.75) -> (-49.62, -5.75)
  line L86 (-49.62, -5.75) -> (-49.62, -7)
  line L87 (-49.62, -7) -> (-47.8702, -7)
  arc A1 (-47.87, -8.5) -> (-47.8702, -7) centre (-47.87, -7.75) ccw
  line L88 (-47.87, -8.5) -> (-49.62, -8.5)
  line L89 (-49.62, -8.5) -> (-49.62, -10)
  line L90 (-49.62, -10) -> (0, -10)
  line L91 (0, -10) -> (0, -8.5)
  line L92 (0, -8.5) -> (-1.75, -8.5)
  arc A2 (-1.75, -7) -> (-1.75, -8.5) centre (-1.75, -7.75) ccw
  line L93 (-1.75, -7) -> (0, -7)
  line L94 (0, -7) -> (0, -5.75)
  line L95 (0, -5.75) -> (-1.7501, -5.75)
  arc A3 (-1.75, -4.25) -> (-1.7501, -5.75) centre (-1.75, -5) ccw
  line L96 (-1.75, -4.25) -> (0, -4.25)
  line L97 (0, -4.25) -> (0, -3)
  line L98 (0, -3) -> (-1.75, -3)
  arc A4 (-1.75, -1.5) -> (-1.75, -3) centre (-1.75, -2.25) ccw
  line L99 (-1.75, -1.5) -> (0, -1.5)
  line L100 (0, -1.5) -> (0, 0)
  line L101 (0, 0) -> (-49.62, 0)
  line L102 (-49.62, 0) -> (-49.62, -1.5)
  line L103 (-49.62, -1.5) -> (-47.87, -1.5)
  arc A5 (-47.87, -3) -> (-47.87, -1.5) centre (-47.87, -2.25) ccw
  line L104 (-47.87, -3) -> (-49.62, -3)
  line L105 (-49.62, -3) -> (-49.62, -4.25)
  line L106 (-10.97, -5) -> (-22.11, -5) construction
  line L107 (-16.54, -5) -> (-16.54, -4.2) construction
  line L108 (-16.54, -5) -> (-16.54, -5.8) construction
  line L109 (-16.54, -5.8) -> (-16.14, -5.8)
  line L110 (-16.54, -5.8) -> (-16.94, -5.8)
  line L111 (-16.94, -5.8) -> (-16.94, -4.2)
  line L112 (-16.94, -4.2) -> (-16.14, -4.2)
  line L113 (-16.14, -4.2) -> (-16.14, -5.8)
  line L114 (-16.14, -5.8) -> (-16.14, -5.5)
  line L115 (-16.14, -4.2) -> (-16.14, -4.5)
  line L116 (-16.14, -4.5) -> (-16.94, -4.5)
  line L117 (-16.14, -5.5) -> (-16.94, -5.5)
  line L118 (-27.51, -5) -> (-38.65, -5) construction
  line L119 (-33.08, -5) -> (-27.51, -5) construction
  line L120 (-30.295, -5) -> (-30.295, -4.2) construction
  line L121 (-30.295, -5) -> (-30.295, -5.8) construction
  line L122 (-33.08, -5) -> (-38.65, -5) construction
  line L123 (-35.865, -5) -> (-35.865, -4.2) construction
  line L124 (-35.865, -5) -> (-35.865, -5.8) construction
  line L125 (-30.295, -5.8) -> (-30.695, -5.8) construction
  line L126 (-30.695, -5.8) -> (-29.895, -5.8)
  line L127 (-29.895, -5.8) -> (-29.895, -4.2)
  line L128 (-29.895, -4.2) -> (-30.695, -4.2)
  line L129 (-30.695, -4.2) -> (-30.695, -5.8)
  line L130 (-35.865, -4.2) -> (-36.265, -4.2) construction
  line L131 (-36.265, -4.2) -> (-36.265, -5.8)
  line L132 (-36.265, -5.8) -> (-35.465, -5.8)
  line L133 (-35.465, -5.8) -> (-35.465, -4.2)
  line L134 (-35.465, -4.2) -> (-36.265, -4.2)
  line L135 (-29.895, -4.2) -> (-29.895, -4.5) construction
  line L136 (-29.895, -5.8) -> (-29.895, -5.5) construction
  line L137 (-29.895, -5.5) -> (-36.265, -5.5)
  line L138 (-29.895, -4.5) -> (-36.265, -4.5)
  dimension "d91" = 0.8
  dimension "d92" = 0.8
  dimension "d93" = 0.4
  dimension "d94" = 0.4
  dimension "d95" = 1.6
  dimension "d96" = 0.8
  dimension "d97" = 0.3
  dimension "d98" = 0.3
  dimension "d103" = 0.8
  dimension "d104" = 0.8
  dimension "d105" = 0.8
  dimension "d106" = 0.8
  dimension "d107" = 0.4
  dimension "d108" = 0.8
  dimension "d109" = 1.6
  dimension "d110" = 0.8
  dimension "d111" = 0.4
  dimension "d112" = 0.8
  dimension "d113" = 1.6
  dimension "d114" = 0.8
  dimension "d115" = 0.3
  constraint midpoint L1 L106.start
  constraint midpoint L45 L106.end
  constraint midpoint L106 L107.start
  constraint perpendicular L106 L107
  constraint perpendicular L106 L108
  constraint perpendicular L108 L109
  constraint perpendicular L108 L110
  constraint perpendicular L110 L111
  constraint perpendicular L107 L112
  constraint perpendicular L109 L114
  constraint perpendicular L112 L115
  constraint coincident L111 L116.end
  constraint perpendicular L111 L116
  constraint coincident L111 L117.end
  constraint perpendicular L111 L117
  constraint midpoint L31 L118.start
  constraint midpoint L65 L118.end
  constraint midpoint L118 L119.start
  constraint midpoint L119 L120.start
  constraint perpendicular L119 L120
  constraint perpendicular L119 L121
  constraint midpoint L122 L123.start
  constraint perpendicular L122 L123
  constraint perpendicular L122 L124
  constraint perpendicular L121 L125
  constraint parallel L125 L126
  constraint perpendicular L126 L127
  constraint perpendicular L127 L128
  constraint perpendicular L123 L130
  constraint perpendicular L130 L131
  constraint perpendicular L124 L132
  constraint perpendicular L132 L133
  constraint perpendicular L131 L134
  constraint perpendicular L128 L135
  constraint vertical L136
  constraint coincident L131 L137.end
  constraint perpendicular L131 L137
  constraint coincident L131 L138.end
  constraint perpendicular L131 L138
  measures "d91" distance of L107.start L107.end
  measures "d92" distance of L107.start L108.end
  measures "d93" distance of L108.end L109.end
  measures "d94" distance of L108.end L110.end
  measures "d95" distance of L110.end L111.end
  measures "d96" distance of L111.end L112.end
  measures "d97" distance of L109.end L114.end
  measures "d98" distance of L112.end L115.end
  measures "d103" distance of L120.start L120.end
  measures "d104" distance of L120.start L121.end
  measures "d105" distance of L123.start L123.end
  measures "d106" distance of L123.start L124.end
  measures "d107" distance of L121.end L125.end
  measures "d108" distance of L125.end L126.end
  measures "d109" distance of L126.end L127.end
  measures "d110" distance of L127.end L128.end
  measures "d111" distance of L123.end L130.end
  measures "d112" distance of L131.end L132.end
  measures "d113" distance of L132.end L133.end
  measures "d114" distance of L133.end L130.end
  measures "d115" distance of L127.end L135.end
extrude "Extrude10" add sketch "Sketch14" along normal blind 0.35 contours L109 L110 L111 L113 L114 L117 | L111 L112 L113 L115 L116 | L126 L127 L129 L137 | L127 L128 L129 L138 | L131 L132 L133 L137 | L131 L133 L134 L138 bodies 1
extrude "Extrude9" add sketch "Sketch14" along normal blind 0.4 contours L111 L113 L116 L117 | L127 L129 L137 L138 | L131 L133 L137 L138 bodies 1
other "Base Mesh Feature1" in component "Component"
other "Modify1" in component "Component"
other "CopyPasteMeshes1" in component "Component"
other "Modify2" in component "Component"
other "Modify3" in component "Component"
component "Component" placed x (1, 0, 0) y (0, 1, 0) z (0, 0, 1) at (0, 0, 0)
